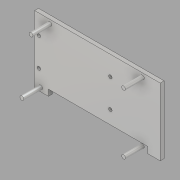
# Autodesk Inventor part: Camera&Pi Holder
Saved by Autodesk Inventor 2017 (Build 210142000, 142)
## iProperties
Created: 2013-12-11
Part Number: Camera&Pi Holder
Material: Aluminum 6061-AHC
Description: STEP AP203
Document SubType Name: Modeling
Designer: qupec
Density: 2.7 g/cm^3
Appearance: Aluminum - Dark
Mass: 25.0409 g
Surface Area: 67.6768 cm^2
Volume: 9.2744 cm^3
Sending System: SolidWorks 2013
Preprocessor: SwSTEP 2.0
Title: ArduinoMega_STEP_AP203.STEP
Revision Number: ANY
Autodesk Inventor part; units mm, degrees
ref_plane "Work Plane10" through (-47.244, -26.7081, 1.651) normal (0, 0, 1) x (1, 0, 0)
sketch "Sketch1" plane through (-47.244, -26.7081, 1.651) normal (0, 0, 1) x (1, 0, 0)
  circle A0 centre (1.2954, 2.54) radius 1.5621 projected
  circle A1 centre (8.7884, 50.8762) radius 1.5621 projected
  circle A2 centre (32.2961, 35.4347) radius 1.3153 projected
  circle A3 centre (32.2961, 7.4185) radius 1.5621 projected
  circle A4 centre (83.9216, 2.54) radius 1.5621 projected
  circle A5 centre (83.9216, 50.8762) radius 1.5621 projected
  line L0 (0, 0) -> (96.52, 0) projected
  line L1 (96.52, 53.4162) -> (0.7474, 53.4162) projected
  line L2 (-3.556, 38.1762) -> (-3.556, 3.556) projected
  line L3 (98.044, 1.524) -> (98.044, 51.8922) projected
  line L4 (98.044, 53.4162) -> (-3.556, 53.4162)
  line L5 (-3.556, 53.4162) -> (-3.556, 0)
  line L6 (-3.556, 0) -> (98.044, 0)
  line L7 (98.044, 0) -> (98.044, 53.4162)
  circle A6 centre (83.9216, 50.8762) radius 1.5621
  circle A7 centre (83.9216, 2.54) radius 1.5621
  circle A8 centre (32.2961, 7.4185) radius 1.5621
  circle A9 centre (32.2961, 35.4347) radius 1.3153
  circle A10 centre (8.7884, 50.8762) radius 1.5621
  circle A11 centre (1.2954, 2.54) radius 1.5621
  point P0 (47.244, 26.7081)
  dimension "d0" = 31.0007
  dimension "d1" = 48.3362
  dimension "d2" = 28.0162
  dimension "d3" = 53.4162
  dimension "d4" = 48.3362
  dimension "d5" = 101.6
  dimension "d6" = 3.1242
  dimension "d7" = 3.1242
  dimension "d8" = 3.1242
  dimension "d9" = 3.1242
  dimension "d10" = 3.1242
  dimension "d11" = 2.6305
  dimension "d12" = 2.54
  dimension "d13" = 12.3444
  dimension "d14" = 2.54
  dimension "d15" = 4.8514
  dimension "d16" = 2.54
  dimension "d17" = 14.1224
  dimension "d18" = 2.54
  dimension "d19" = 14.1224
  dimension "d67" = 101.6
  dimension "d68" = 53.4162
  constraints: 8 end point, 6 centre point, 6 coincident, 6 concentric, 2 parallel, 1 horizontal, 1 perpendicular, 1 point on line
  measures "d0" horizontal distance of A3.centre A0.centre
  measures "d1" vertical distance of A1.centre A0.centre
  measures "d2" distance of A2.centre A3.centre
  measures "d3" distance between parallel lines of L1 L0
  measures "d4" distance of A5.centre A4.centre
  measures "d5" distance between parallel lines of L3 L2
  measures "d6" diameter of A3
  measures "d7" diameter of A0
  measures "d8" diameter of A1
  measures "d9" diameter of A4
  measures "d10" diameter of A5
  measures "d11" diameter of A2
  measures "d12" distance from line of L1 A1.centre
  measures "d13" distance from line of L2 A1.centre
  measures "d14" distance from line of L0 A0.centre
  measures "d15" distance from line of L2 A0.centre
  measures "d16" distance from line of L1 A5.centre
  measures "d17" distance from line of L3 A5.centre
  measures "d18" distance from line of L0 A4.centre
  measures "d19" distance from line of L3 A4.centre
  measures "d67" distance between parallel lines of L2 L7
  measures "d68" distance of L4.end L5.end
ref_plane "Work Plane2" through (-47.244, -26.7081, 1.651) normal (0, 0, 1) x (1, 0, 0)
sketch "Sketch2" plane through (-47.244, -26.7081, 1.651) normal (0, 0, 1) x (1, 0, 0)
  circle A0 centre (71.8216, 83.8772) radius 1.5621
  circle A1 centre (64.3286, 35.541) radius 1.5621
  circle A2 centre (146.9548, 35.541) radius 1.5621
  circle A3 centre (146.9548, 83.8772) radius 1.5621
  line L0 (115.9668, 75.089) -> (64.3286, 75.089) construction
  line L1 (115.9668, 33.001) -> (64.3286, 33.001) construction
  dimension "d98" = 3.1242
  dimension "d99" = 3.1242
  dimension "d100" = 3.1242
  dimension "d101" = 3.1242
  dimension "d102" = 82.6262
  dimension "d104" = 0
  dimension "d105" = 48.3362
  dimension "d130" = 2.54
  dimension "d131" = 2.54
  dimension "d132" = 75.1332
  dimension "d133" = 48.3362
  constraints: 4 centre point, 4 end point, 2 horizontal
  measures "d98" diameter of A3
  measures "d99" diameter of A0
  measures "d100" diameter of A1
  measures "d101" diameter of A2
  measures "d102" distance of A2.centre A1.centre
  measures "d104" horizontal distance of A2.centre A3.centre
  measures "d105" distance of A2.centre A3.centre
  measures "d130" distance from line of L1 A2.centre
  measures "d131" distance from line of L1 A1.centre
  measures "d132" distance of A3.centre A0.centre
  measures "d133" vertical distance of A1.centre A0.centre
ref_plane "Work Plane3" through (-14.9479, -19.2896, -20.574) normal (0, 0, -1) x (-1, 0, 0)
sketch "Sketch3" plane through (-14.9479, -19.2896, -20.574) normal (0, 0, -1) x (-1, 0, 0)
  line L0 (12.7, -3.175) -> (-48.4505, -3.175)
  line L1 (-48.4505, 31.1912) -> (12.7, 31.1912)
  line L2 (12.7, 31.1912) -> (12.7, -3.175)
  line L3 (-54.8005, 45.9977) -> (-48.4505, 45.9977)
  line L4 (-48.4505, 45.9977) -> (-48.4505, 31.1912)
  line L5 (-48.4505, -3.175) -> (-48.4505, -7.4185)
  line L6 (-48.4505, -7.4185) -> (-54.8005, -7.4185)
  circle A0 centre (0, 0) radius 1.5621 construction
  circle A1 centre (0, 28.0162) radius 1.3153 construction
  circle A2 centre (-51.6255, 43.4577) radius 1.5621 construction
  circle A3 centre (-51.6255, -4.8785) radius 1.5621 construction
  line L7 (-54.8005, -7.4185) -> (-54.8005, 45.9977)
  line L8 (-64.2239, 45.9977) -> (31.5487, 45.9977) projected
  line L9 (32.2961, -7.4185) -> (-64.2239, -7.4185) projected
  point P0 (-14.9479, 19.2896)
  point P1 (0, 14.0081)
  point P2 (-25.8127, 14.0081)
  dimension "d24" = 28.0162
  dimension "d25" = 14.0081
  dimension "d26" = 17.1831
  dimension "d29" = 51.6255
  dimension "d30" = 25.8128
  dimension "d36" = 3.175
  dimension "d37" = 3.175
  dimension "d38" = 3.175
  dimension "d39" = 0
  dimension "d40" = 0
  dimension "d41" = 3.175
  dimension "d48" = 12.7
  constraints: 16 end point, 4 perpendicular, 1 horizontal, 1 parallel, 1 point on line, 1 vertical
  measures "d24" distance of A1.centre A0.centre
  measures "d25" distance of A0.centre point (0, 14.008)
  measures "d26" distance from line of point (0, 14.008) L1
  measures "d29" horizontal distance of A3.centre A0.centre
  measures "d30" horizontal distance of point (-25.813, 14.008) A0.centre
  measures "d36" distance from line of L0 A0.centre
  measures "d37" distance from line of A1.centre L1
  measures "d38" distance from line of L7 A3.centre
  measures "d39" distance between parallel lines of L3 L8
  measures "d40" distance between parallel lines of L9 L6
  measures "d41" distance from line of A2.centre L4
  measures "d48" distance from line of L2 A0.centre
extrude "Extrusion3" [suppressed]
ref_plane "Work Plane4" through (-47.244, -26.7081, 1.651) normal (0, 0, 1) x (1, 0, 0)
ref_plane "Work Plane8" through (57.15, 17.5006, -10.795) normal (0, 0, -1) x (-1, 0, 0)
ref_plane "Work Plane9" through (52.6288, -22.8981, 0) normal (1, 0, 0) x (0, 0, -1)
extrude "Extrusion12" add sketch "Sketch2" along normal blind 15.24
sketch "Sketch18" plane through (99.7108, 57.1691, 1.651) normal (0, 0, -1) x (-1, 0, 0)
  line L0 (6.35, 3.175) -> (-14.478, 3.175)
  line L1 (-14.478, 3.175) -> (-14.478, -51.5112)
  line L2 (-14.478, -51.5112) -> (6.35, -51.5112)
  line L3 (6.35, -51.5112) -> (6.35, 3.175)
  circle A0 centre (0, 0) radius 1.5621 construction
  circle A1 centre (0, -48.3362) radius 1.5621 construction
  line L4 (0, 0) -> (0, -48.3362) construction
  line L5 (6.35, 3.175) -> (87.4776, 3.175)
  line L6 (87.4776, 3.175) -> (87.4776, -51.5112)
  line L7 (87.4776, -51.5112) -> (6.35, -51.5112)
  line L8 (6.35, -51.5112) -> (6.35, 3.175)
  circle A2 centre (75.1332, 0) radius 1.5621 construction
  circle A3 centre (82.6262, -48.3362) radius 1.5621 projected
  line L9 (0, -48.3362) -> (82.6262, -48.3362) construction
  point P0 (99.7108, -57.1691)
  point P1 (0, -24.1681)
  point P2 (41.3131, -48.3362)
  dimension "d116" = 20.828
  dimension "d117" = 14.478
  dimension "d120" = 24.1681
  dimension "d121" = 48.3362
  dimension "d122" = 54.6862
  dimension "d123" = 27.3431
  dimension "d124" = 54.6862
  dimension "d126" = 0
  dimension "d127" = 101.9556
  dimension "d137" = 41.3131
  dimension "d138" = 82.6262
  dimension "d139" = 55.7911
  dimension "d140" = 4.8514
  constraints: 20 end point, 4 parallel, 3 horizontal, 2 midpoint, 2 perpendicular, 1 point on line, 1 vertical
  measures "d116" distance of L1.end L2.end
  measures "d117" distance from line of L4.end L1
  measures "d120" distance of L4.start point (0, -24.168)
  measures "d121" distance of L4.start L4.end
  measures "d122" distance of L0.end L1.end
  measures "d123" distance from line of point (0, -24.168) L0
  measures "d124" distance between parallel lines of L7 L5
  measures "d126" distance between parallel lines of L0 L5
  measures "d127" distance between parallel lines of L6 L1
  measures "d137" distance of L9.end point (41.313, -48.336)
  measures "d138" distance of L4.end L9.end
  measures "d139" distance from line of point (41.313, -48.336) L1
  measures "d140" distance from line of L6 L9.end
extrude "Extrusion13" add sketch "Sketch18" along normal blind 3.175 contours L3 L2 L1 L0 | L5 L6 L7 L3 | A3
sketch "Sketch19" plane through (99.7108, 57.1691, 16.891) normal (0, 0, 1) x (1, 0, 0)
  circle A0 centre (0, 0) radius 1.5621 projected
  circle A1 centre (0, -48.3362) radius 1.5621 projected
  circle A2 centre (-75.1332, 0) radius 1.5621 projected
  circle A3 centre (-82.6262, -48.3362) radius 1.5621 projected
  line L0 (14.478, -51.5112) -> (14.478, 3.175) projected
  point P0 (-99.7108, -57.1691)
  dimension "d134" = 82.6262
  dimension "d135" = 14.478
  measures "d134" distance of A3.centre A1.centre
  measures "d135" distance from line of L0 A1.centre
sketch "Sketch20" plane through (99.7108, 57.1691, -1.524) normal (0, 0, -1) x (-1, 0, 0)
  circle A0 centre (83.9776, -12.6681) radius 1.375
  circle A1 centre (83.9776, -35.6681) radius 1.375
  circle A2 centre (25.9776, -12.6681) radius 1.375
  circle A3 centre (25.9776, -35.6681) radius 1.375
  line L0 (-14.478, 3.175) -> (-14.478, -51.5112) projected
  line L1 (25.9776, -12.6681) -> (25.9776, -35.6681) construction
  line L2 (-14.478, -51.5112) -> (87.4776, -51.5112) projected
  line L3 (87.4776, -51.5112) -> (87.4776, 3.175) projected
  point P0 (99.7108, -57.1691)
  point P1 (25.9776, -24.1681)
  dimension "d141" = 2.75
  dimension "d142" = 2.75
  dimension "d143" = 2.75
  dimension "d144" = 2.75
  dimension "d145" = 23
  dimension "d146" = 23
  dimension "d147" = 58
  dimension "d149" = 11.5
  dimension "d150" = 54.6862
  dimension "d151" = 27.3431
  dimension "d152" = 0
  dimension "d155" = 3.5
  dimension "d156" = 3.5
  constraints: 4 centre point, 2 end point, 1 midpoint, 1 vertical
  measures "d141" diameter of A1
  measures "d142" diameter of A0
  measures "d143" diameter of A2
  measures "d144" diameter of A3
  measures "d145" distance of A1.centre A0.centre
  measures "d146" distance of L1.end L1.start
  measures "d147" distance of A1.centre L1.end
  measures "d149" distance of L1.end point (25.978, -24.168)
  measures "d150" distance of L0.start L0.end
  measures "d151" distance from line of L2 point (25.978, -24.168)
  measures "d152" vertical distance of L1.start A0.centre
  measures "d155" distance from line of A1.centre L3
  measures "d156" distance from line of L3 A0.centre
extrude "Extrusion14" cut sketch "Sketch20" against normal through all
sketch "Sketch21" plane through (99.7108, 57.1691, -1.524) normal (0, 0, -1) x (-1, 0, 0)
  circle A0 centre (0, -48.3362) radius 1.5621 projected
  circle A1 centre (0, -48.3362) radius 1.5621 projected
  circle A2 centre (0, 0) radius 1.5621 projected
  circle A3 centre (0, 0) radius 1.5621 projected
  circle A4 centre (75.1332, 0) radius 1.5621 projected
  circle A5 centre (75.1332, 0) radius 1.5621 projected
  circle A6 centre (82.6262, -48.3362) radius 1.5621 projected
  circle A7 centre (82.6262, -48.3362) radius 1.5621 projected
  line L0 (-14.478, -51.5112) -> (87.4776, -51.5112) projected
  line L1 (-4.318, -51.5112) -> (76.2762, -51.5112)
  line L2 (76.2762, -51.5112) -> (76.2762, -46.4312)
  line L3 (76.2762, -46.4312) -> (-4.318, -46.4312)
  line L4 (-4.318, -46.4312) -> (-4.318, -51.5112)
  line L5 (-14.478, 3.175) -> (-14.478, -51.5112) projected
  point P0 (99.7108, -57.1691)
  dimension "d157" = 6.35
  dimension "d159" = 5.08
  dimension "d162" = 10.16
  constraints: 8 end point, 2 parallel, 1 horizontal, 1 perpendicular, 1 point on line
  measures "d157" distance from line of A6.centre L2
  measures "d159" distance between parallel lines of L0 L3
  measures "d162" distance between parallel lines of L5 L4
extrude "Extrusion15" cut sketch "Sketch21" against normal up to surface (3.175 mm away) contours A0 | L4 L3 L2 L0
equation "\"d25\" = 0.5 * d24"
equation "\"d26\" = 0.5 * d22"
equation "\"d30\" = 0.5 * d29"
equation "\"d37\" = d36"
equation "\"d38\" = d41"
equation "\"d99\" = d98"
equation "\"d100\" = d99"
equation "\"d101\" = d98"
equation "\"d120\" = 0.5 * d121"
equation "\"d123\" = 0.5 * d122"
equation "\"d124\" = d122"
equation "\"d137\" = 0.5 * d138"
equation "\"d142\" = d141"
equation "\"d143\" = d141"
equation "\"d144\" = d141"
equation "\"d149\" = 0.5 * d146"
equation "\"d151\" = 0.5 * d150"
equation "\"d74\" = d71"
equation "\"d71\" = 3.175"
equation "\"d22\" = 34.3662"
body "Solid1"
